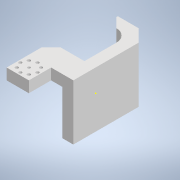
# Autodesk Inventor part: wobble goal arm
Saved by Autodesk Inventor 2020 (Build 240168000, 168)
## iProperties
Created: 2020-09-26
Part Number: wobble goal arm
Material: Generic
Document SubType Name: Modeling
Designer: elois
Density: 1 g/cm^3
Appearance: Default
Author: elois
Autodesk Inventor part; units mm, degrees
ref_plane "YZ Plane" through (0, 0, 0) normal (1, 0, 0) x (0, 1, 0)
ref_plane "XZ Plane" through (0, 0, 0) normal (0, 1, 0) x (-1, 0, 0)
ref_plane "XY Plane" through (0, 0, 0) normal (0, 0, 1) x (1, 0, 0)
sketch "Sketch1" plane through (0, 0, 0) normal (0, 1, 0) x (-1, 0, 0)
  line L0 (0, 0) -> (50.8, 0)
  line L1 (50.8, 0) -> (50.8, -25.4)
  line L2 (50.8, -25.4) -> (0, -25.4)
  line L3 (0, -25.4) -> (0, 0)
  line L4 (25.4, -25.4) -> (25.4, -38.1)
  line L5 (25.4, -38.1) -> (50.8, -38.1)
  line L6 (50.8, -38.1) -> (50.8, -25.4)
  dimension "d0" = 50.8
  dimension "d1" = 25.4
  dimension "d2" = 50.8
  dimension "d3" = 90
  constraints: 14 end point, 2 perpendicular, 2 vertical, 1 horizontal, 1 midpoint
  measures "d0" distance of L0.start L0.end
  measures "d1" distance of L0.end L1.end
  measures "d2" distance of L1.end L2.end
  measures "d3" angle of L1 L2
extrude "Extrusion1" add sketch "Sketch1" along normal blind 12.7
move or copy body "Move Body1" bodies to move or copy 1 copy no rotation origin (0, 0, 0) rotation axis (0, 1, 0) rotation angle -90 translate (-76.2, 0, 25.4)
sketch "Sketch3" plane through (-76.2, 12.7, 25.4) normal (0, 1, 0) x (1, 0, 0)
  point P0 (76.2, 25.4)
sketch "Sketch4" plane through (-76.2, 12.7, 25.4) normal (0, 1, 0) x (1, 0, 0)
  line L0 (25.4, 0) -> (25.4, 25.4) projected
  line L1 (25.4, 12.7) -> (0, 12.7)
  line L2 (0, 50.8) -> (0, 0) projected
  circle A0 centre (12.7, 12.7) radius 9.779
  circle A1 centre (12.7, 12.7) radius 1.5
  circle A2 centre (12.7, 22.479) radius 1.7526
  circle A3 centre (5.7852, 19.6148) radius 1.7526
  circle A4 centre (2.921, 12.7) radius 1.7526
  circle A5 centre (5.7852, 5.7852) radius 1.7526
  circle A6 centre (12.7, 2.921) radius 1.7526
  circle A7 centre (19.6148, 5.7852) radius 1.7526
  circle A8 centre (22.479, 12.7) radius 1.7526
  circle A9 centre (19.6148, 19.6148) radius 1.7526
  point P0 (76.2, 25.4)
  point P1 (25.4, 50.8)
  point P2 (25.4, 19.05)
  dimension "d16" = 19.558
  dimension "d17" = 3
  dimension "d18" = 3.5052
  dimension "d21" = 360
  constraints: 9 centre point, 2 end point, 1 coincident, 1 horizontal, 1 midpoint, 1 point on line, 1 vertical alignment, 19 other
  measures "d17" diameter of A1
  measures "d18" diameter of A2
extrude "Extrusion3" cut sketch "Sketch4" against normal blind 25.4 contours A8 A0 L1 | L1 A0 A8 | A0 A8 L1 | L1 A8 A0 | A9 A0 | A0 A9 | A7 A0 | A0 A7 | A1 L1 | L1 A1 | A2 A0 | A0 A2 | A6 A0 | A0 A6 | A4 A0 L1 | L1 A0 A4 | A0 A4 L1 | L1 A4 A0 | A3 A0 | A0 A3 | A5 A0 | A0 A5
sketch "Sketch6" plane through (-38.1, 0, 0) normal (1, 0, 0) x (0, 0, -1)
  line L0 (25.4, 12.7) -> (-25.4, 12.7) projected
  line L1 (0, 12.7) -> (0, -50.8)
  line L2 (0, -50.8) -> (50.8, -50.8)
  line L3 (50.8, -50.8) -> (50.8, 12.7)
  line L4 (50.8, 12.7) -> (0, 12.7)
  line L5 (50.8, 12.7) -> (76.2, 12.7)
  line L6 (76.2, 12.7) -> (76.2, -50.8)
  line L7 (76.2, -50.8) -> (50.8, -50.8)
  point P0 (0, 0)
  dimension "d33" = 63.5
  dimension "d34" = 50.8
  dimension "d37" = 25.4
  constraints: 14 end point, 4 perpendicular, 1 collinear, 1 horizontal, 1 midpoint, 1 vertical
  measures "d33" distance of L1.start L1.end
  measures "d34" distance of L1.end L2.end
  measures "d37" distance of L3.end L5.end
extrude "Extrusion5" add sketch "Sketch6" along normal blind 12.7
sketch "Sketch9" plane through (-38.1, -50.8, -76.2) normal (0, 0, -1) x (-1, 0, 0)
  line L0 (12.7, 63.5) -> (-12.7, 63.5) projected
  line L1 (-12.7, 63.5) -> (25.4, 63.5)
  line L2 (38.1, 63.5) -> (12.7, 63.5) projected
  line L3 (25.4, 63.5) -> (25.4, 0)
  line L4 (25.4, 0) -> (-12.7, 0)
  line L5 (-12.7, 0) -> (-12.7, 63.5)
  point P0 (-38.1, 50.8)
  dimension "d39" = 63.5
  constraints: 8 end point, 2 perpendicular, 1 midpoint, 1 vertical
  measures "d39" distance of L1.end L3.end
extrude "Extrusion6" add sketch "Sketch9" along normal blind 12.7
chamfer "Chamfer1" distance 14.2875 angle 45 1 edges at (-25.4, -19.05, -88.9)
chamfer "Chamfer2" distance 11.1125 angle 45 1 edges at (-63.5, -19.05, -76.2)
chamfer "Chamfer3" distance 11.1125 angle 45 1 edges at (-76.2, 6.35, -25.4)
fillet "Fillet1" radius 14.2875 1 edges at (-38.1, -19.05, -76.2)
body "Solid1"
